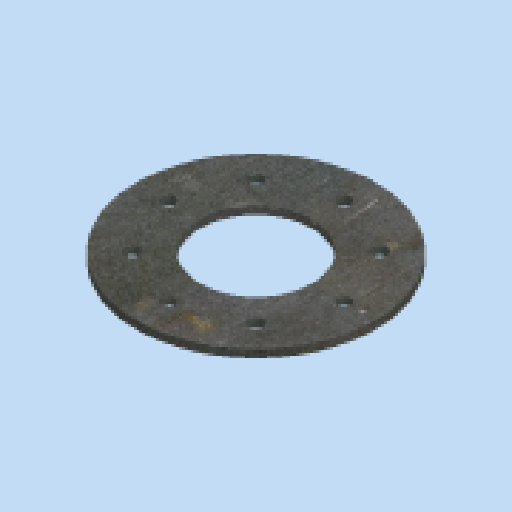
# Autodesk Inventor part: plateHole
Saved by Autodesk Inventor 2023 (Build 270158000, 158)
## iProperties
Created: 2026-04-08
Part Number: plateHole
Material: Steel
Document SubType Name: Modeling
Designer: Nathann
Density: 7.85 g/cm^3
Appearance: Plate
Author: Nathann
Autodesk Inventor part; units mm, degrees
ref_plane "YZ Plane" through (0, 0, 0) normal (1, 0, 0) x (0, 1, 0)
ref_plane "XZ Plane" through (0, 0, 0) normal (0, 1, 0) x (-1, 0, 0)
ref_plane "XY Plane" through (0, 0, 0) normal (0, 0, 1) x (1, 0, 0)
sketch "Sketch1" plane through (0, 0, 0) normal (0, 1, 0) x (-1, 0, 0)
  circle A0 centre (0, 0) radius 75
  circle A1 centre (0, 0) radius 35
  circle A2 centre (55, 0) radius 4.25
  circle A3 centre (38.8909, 38.8909) radius 4.25
  circle A4 centre (0, 55) radius 4.25
  circle A5 centre (-38.8909, 38.8909) radius 4.25
  circle A6 centre (-55, 0) radius 4.25
  circle A7 centre (-38.8909, -38.8909) radius 4.25
  circle A8 centre (0, -55) radius 4.25
  circle A9 centre (38.8909, -38.8909) radius 4.25
  dimension "d0" = 150
  dimension "d1" = 70
  dimension "d2" = 55
  dimension "d3" = 8.5
  dimension "d6" = 360
  constraints: 10 centre point, 2 coincident, 17 other
  measures "d0" diameter of A0
  measures "d1" diameter of A1
  measures "d2" distance of A2.centre point (0, 0)
  measures "d3" diameter of A2
extrude "Extrusion1" add sketch "Sketch1" along normal blind 5
body "Solid1"
